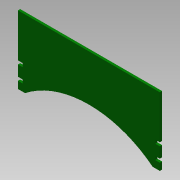
# Autodesk Inventor part: 104_CellScopeDomeBoard_v3
Saved by Autodesk Inventor 2015 (Build 190159000, 159)
## iProperties
Created: 2014-07-14
Part Number: 104_CellScopeDomeBoard_v3
Material: Generic
Document SubType Name: Modeling
Designer: Zack
Density: 1 g/cm^3
Appearance: Default
Author: Zack
Autodesk Inventor part; units mm, degrees
ref_plane "YZ Plane" through (0, 0, 0) normal (1, 0, 0) x (0, 1, 0)
ref_plane "XZ Plane" through (0, 0, 0) normal (0, 1, 0) x (-1, 0, 0)
ref_plane "XY Plane" through (0, 0, 0) normal (0, 0, 1) x (1, 0, 0)
sketch "Sketch2" plane through (0, 0, 0) normal (0, 0, 1) x (1, 0, 0)
  arc A0 (44.975, 57.5) -> (-44.975, 57.5) centre (0, 0) ccw
  line L0 (-70, 0) -> (70, 0) projected
  line L1 (-50, 105.5) -> (50, 105.5)
  line L2 (-50, 57.5) -> (-44.975, 57.5)
  line L3 (44.975, 57.5) -> (50, 57.5)
  line L4 (-50, 75) -> (-47, 75)
  line L5 (-46.75, 74.75) -> (-46.75, 72.75)
  line L6 (-47, 72.5) -> (-50, 72.5)
  line L7 (-50, 65) -> (-47, 65)
  line L8 (-46.75, 64.75) -> (-46.75, 62.75)
  line L9 (-47, 62.5) -> (-50, 62.5)
  line L10 (-50, 105.5) -> (-50, 75)
  line L11 (-50, 72.5) -> (-50, 65)
  line L12 (-50, 62.5) -> (-50, 57.5)
  arc A1 (-46.75, 74.75) -> (-47, 75) centre (-47, 74.75) ccw
  arc A2 (-47, 72.5) -> (-46.75, 72.75) centre (-47, 72.75) ccw
  arc A3 (-46.75, 64.75) -> (-47, 65) centre (-47, 64.75) ccw
  arc A4 (-47, 62.5) -> (-46.75, 62.75) centre (-47, 62.75) ccw
  line L13 (0, -21.1) -> (0, 126.6) projected
  line L14 (50, 75) -> (47, 75)
  line L15 (46.75, 74.75) -> (46.75, 72.75)
  line L16 (47, 72.5) -> (50, 72.5)
  line L17 (50, 65) -> (47, 65)
  line L18 (46.75, 64.75) -> (46.75, 62.75)
  line L19 (47, 62.5) -> (50, 62.5)
  line L20 (50, 72.5) -> (50, 65)
  arc A5 (47, 75) -> (46.75, 74.75) centre (47, 74.75) ccw
  arc A6 (46.75, 72.75) -> (47, 72.5) centre (47, 72.75) ccw
  arc A7 (47, 65) -> (46.75, 64.75) centre (47, 64.75) ccw
  arc A8 (46.75, 62.75) -> (47, 62.5) centre (47, 62.75) ccw
  line L21 (50, 75) -> (50, 105.5)
  line L22 (50, 57.5) -> (50, 62.5)
  line L23 (50, 65) -> (50, 72.5)
  point P0 (50, 55.9017)
  point P1 (-50, 55.9017)
  point P2 (0.9884, 19.8204)
  dimension "d0" = 73
  dimension "d33" = 100
  dimension "d34" = 211
  dimension "d37" = 115
  dimension "d38" = 2.5
  dimension "d39" = 2.5
  dimension "d41" = 0.25
  dimension "d42" = 3.25
  dimension "d43" = 5
  dimension "d44" = 10
  constraints: 46 end point, 18 point on circle, 16 symmetric about line, 11 perpendicular, 9 centre point, 9 parallel, 8 tangent, 4 collinear, 4 horizontal, 3 equal radius, 3 vertical, 1 coincident, 1 horizontal alignment, 4 other
  measures "d0" radius of A0
  measures "d33" distance of L1.start L1.end
  measures "d34" diameter of L1 L0
  measures "d37" diameter of L2 L0
  measures "d38" distance between parallel lines of L6 L4
  measures "d39" distance between parallel lines of L9 L7
  measures "d41" radius of A1
  measures "d42" distance between parallel lines of L11 L8
  measures "d43" distance between parallel lines of L2 L9
  measures "d44" distance between parallel lines of L6 L9
extrude "Extrusion4" add sketch "Sketch2" along normal mid plane 1.57
body "Solid4"
